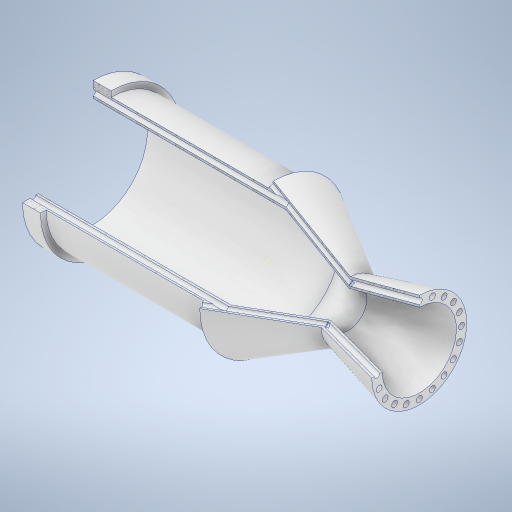
# Autodesk Inventor part: aluminium engine
Saved by Autodesk Inventor 2023 (Build 270158000, 158)
## iProperties
Created: 2022-09-15
Part Number: aluminium engine
Material: Aluminum 6061
Document SubType Name: Modeling
Designer: station
Density: 2.7 g/cm^3
Appearance: Aluminum - Flat
Author: station
Autodesk Inventor part; units mm, degrees
ref_plane "XZ Plane" through (0, 0, 0) normal (0, 1, 0) x (-1, 0, 0)
sketch "Sketch2" plane through (0, 0, 0) normal (0, 0, 1) x (1, 0, 0)
  line L0 (0, 54.5) -> (192, 54.5)
  line L1 (254.7886, 18.124) -> (254.7886, 0) construction
  line L2 (192, 54.5) -> (254.7886, 18.124)
  line L3 (254.7886, 18.124) -> (325.1228, 36.97)
  line L4 (254.7886, 18.124) -> (254.7886, 43.3259) construction
  line L5 (0, 0) -> (254.7886, 0)
  line L6 (325.1228, 36.97) -> (325.1228, 0)
  line L7 (0, 64.5) -> (174.6795, 64.5)
  line L8 (194.6795, 64.375) -> (256.2014, 28.8553)
  line L9 (256.2014, 28.8553) -> (325.1228, 47.3228)
  line L10 (325.1228, 36.97) -> (325.1228, 47.3228)
  line L11 (0, 54.5) -> (0, 64.5)
  line L12 (174.6795, 64.5) -> (164.6795, 64.5)
  line L13 (174.6795, 64.5) -> (179.6254, 73.0665)
  line L14 (194.6795, 64.375) -> (179.6254, 73.0665)
  line L15 (0, 0) -> (0, 70)
  line L16 (0, 70) -> (18, 70)
  line L17 (18, 70) -> (18, 64.5)
  line L18 (192, 54.5) -> (254.7886, 18.124)
  line L19 (194.5065, 58.8264) -> (257.295, 22.4504)
  line L20 (194.5065, 58.8264) -> (139.8332, 90.392)
  point P0 (254.7886, 31.9804)
  point P1 (0, 64.375)
  dimension "d2" = 18.124
  dimension "d9" = 54.5
  dimension "d43" = 192
  dimension "d44" = 10
  dimension "d45" = 10
  dimension "d47" = 60
  dimension "d48" = 70
  dimension "d49" = 18
  dimension "d69" = 5
  constraints: 42 end point, 5 vertical, 3 point on line, 2 parallel, 2 perpendicular, 1 collinear
  measures "d2" distance of L1.start L1.end
  measures "d9" distance from line of L5.start L0
  measures "d43" distance of L0.start L0.end
  measures "d44" distance between parallel lines of L0 L7
  measures "d45" distance of L7.end L12.end
  measures "d47" angle of L7 L13
  measures "d48" distance of L5.start L15.end
  measures "d49" distance of L15.end L16.end
  measures "d69" distance between parallel lines of L2 L19
revolve "Revolution1" add sketch "Sketch2" angle 360 about axis through (0, 0, 0) along (1, 0, 0)
sketch "Sketch9" plane through (0, 0, 0) normal (-1, 0, 0) x (0, 0, 1)
  circle A0 centre (0, 0) radius 59.5 construction
  circle A1 centre (0, 59.5) radius 3
  dimension "d50" = 119
  dimension "d51" = 6
  constraints: 1 centre point, 1 coincident, 1 vertical alignment, 2 other
  measures "d51" diameter of A1
extrude "Extrusion2" cut sketch "Sketch9" against normal blind 192
pattern_circular "Circular Pattern1" count 20 over 360 about axis through (-10, 0, 0) along (1, 0, 0) of "Extrusion2"
ref_plane "Work Plane7" through (175, 0, 0) normal (1, 0, 0) x (0, 1, 0)
sketch "Sketch11" plane through (175, 0, 0) normal (1, 0, 0) x (0, 1, 0)
  point P0 (0, 0)
sketch "Sketch13" plane through (325.1228, 0, 0) normal (1, 0, 0) x (0, 0, -1)
  circle A0 centre (0, 0) radius 42
  circle A1 centre (0, 42) radius 3
  dimension "d58" = 84
  dimension "d59" = 6
  constraints: 1 centre point, 1 coincident, 1 vertical alignment, 2 other
  measures "d59" diameter of A1
ref_plane "Work Plane8" through (0, 0, 0) normal (0, 0, 1) x (1, 0, 0)
sketch "Sketch14" plane through (0, 0, 0) normal (0, 0, 1) x (1, 0, 0)
  line L0 (325.1228, -47.3228) -> (325.1228, 47.3228) projected
  line L1 (325.1228, 42.329) -> (254.5849, 23.4284)
  line L2 (256.2014, 28.8553) -> (325.1228, 47.3228) projected
  point P0 (0, 0)
  constraints: 2 end point, 1 parallel, 1 point on line
sweep "Sweep2" cut profiles "Sketch13" path "Sketch14" picked at (-0.1178, 40.999) picked at (0.1042, 42.9866) path curves L1 contours A1 A0 | A0 A1
pattern_circular "Circular Pattern2" count 20 over 360 about axis through (-10, 0, 0) along (1, 0, 0) of "Sweep2"
sketch "Sketch15" plane through (175, 0, 0) normal (1, 0, 0) x (0, 1, 0)
  point P0 (0, 0)
ref_plane "Work Plane12" through (103.057, -59.5, 0) normal (-0.8660254, 0.5, 0) x (0, 0, 1)
ref_plane "Work Plane11" through (0, 0, 0) normal (-0.8660254, 0.5, 0) x (0, 0, 1)
sketch "Sketch16" plane through (103.057, -59.5, 0) normal (-0.8660254, 0.5, 0) x (0, 0, 1)
  point P0 (0, 0)
sketch "Sketch17" plane through (103.057, -59.5, 0) normal (-0.8660254, 0.5, 0) x (0, 0, 1)
  circle A0 centre (0, 148.1254) radius 3
  point P0 (0, 0)
  dimension "d70" = 6
  constraints: 1 centre point
  measures "d70" diameter of A0
extrude "Extrusion3" cut sketch "Sketch17" against normal blind 93
pattern_circular "Circular Pattern3" count 20 over 360 about axis through (-10, 0, 0) along (1, 0, 0) of "Extrusion3"
body "Solid1"
